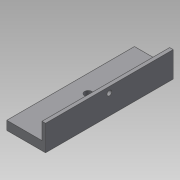
# Autodesk Inventor part: Угольник
Saved by Autodesk Inventor 2014 SP1 (Build 180222100, 222)
## iProperties
Created: 2014-04-11
Part Number: Угольник
Material: Типовые
Document SubType Name: Modeling
Designer: Украинцев
Mass: 593.26 g
Surface Area: 895.086 cm^2
Volume: 593.26 cm^3
Density: 1 g/cm^3
Appearance: По умолчанию
Author: Украинцев
Autodesk Inventor part; units mm, degrees
ref_plane "YZ Plane" through (0, 0, 0) normal (1, 0, 0) x (0, 1, 0)
ref_plane "XZ Plane" through (0, 0, 0) normal (0, 1, 0) x (-1, 0, 0)
ref_plane "XY Plane" through (0, 0, 0) normal (0, 0, 1) x (1, 0, 0)
sketch "Эскиз1" plane through (0, 0, 0) normal (0, 0, 1) x (1, 0, 0)
  line L0 (-44, 145) -> (44, 145)
  line L1 (44, 145) -> (44, -145)
  line L2 (44, -145) -> (-44, -145)
  line L3 (-44, -145) -> (-44, 145)
  line L4 (-44, 145) -> (44, -145) construction
  line L5 (44, 145) -> (-44, -145) construction
  circle A0 centre (-4, 0) radius 8.5
  point P0 (0, 0)
  dimension "d0" = 88
  dimension "d1" = 290
  dimension "d2" = 17
  dimension "d3" = 40
  dimension "d4" = 145
  constraints: 12 end point, 2 midpoint, 2 parallel, 1 centre point, 1 horizontal, 1 perpendicular
  measures "d0" distance of L1.end L2.end
  measures "d1" distance of L0.end L1.end
  measures "d2" diameter of A0
  measures "d3" distance from line of A0.centre L3
  measures "d4" distance from line of A0.centre L2
extrude "Выдавливание1" add sketch "Эскиз1" along normal mid plane 20
sketch "Эскиз2" plane through (44, -145, 10) normal (1, 0, 0) x (0, 0, -1)
  line L0 (20, 290) -> (20, 0) projected
  line L1 (20, 290) -> (-38, 290)
  line L2 (-38, 290) -> (-38, 0)
  line L3 (-38, 0) -> (20, 0)
  line L4 (20, 0) -> (20, 290)
  circle A0 centre (-25, 145) radius 5.5
  line L5 (0, 0) -> (0, 290) projected
  point P0 (10, 145)
  dimension "d7" = 58
  dimension "d8" = 11
  dimension "d9" = 25
  dimension "d10" = 145
  constraints: 8 end point, 2 parallel, 1 centre point, 1 horizontal, 1 perpendicular
  measures "d7" distance of L0.start L1.end
  measures "d8" diameter of A0
  measures "d9" distance from line of A0.centre L5
  measures "d10" distance from line of A0.centre L3
extrude "Выдавливание2" add sketch "Эскиз2" against normal blind 8
